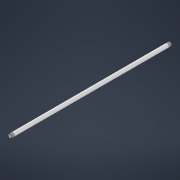
# Autodesk Inventor part: Welle
Saved by Autodesk Inventor 2021 (Build 250183000, 183)
## iProperties
Created: 2023-10-25
Part Number: Welle
Material: Generisch
Document SubType Name: Modeling
Designer: Tobias Sauter
Density: 1 g/cm^3
Appearance: Vorgabe
Author: Team 8
Autodesk Inventor part; units mm, degrees
ref_plane "YZ Plane" through (0, 0, 0) normal (1, 0, 0) x (0, 1, 0)
ref_plane "XZ Plane" through (0, 0, 0) normal (0, 1, 0) x (-1, 0, 0)
ref_plane "XY Plane" through (0, 0, 0) normal (0, 0, 1) x (1, 0, 0)
sketch "Skizze1" plane through (0, 0, 0) normal (0, 0, 1) x (1, 0, 0)
  circle A0 centre (0, 0) radius 2.5
  dimension "d0" = 5
  constraints: 1 centre point, 1 coincident
  measures "d0" diameter of A0
extrude "Extrusion1" add sketch "Skizze1" along normal blind 215
thread "Gewinde1" size "M5x0.8" class "6g" standard "ISO Metric profile" length 4.2
thread "Gewinde2" size "M5x0.8" class "6g" standard "ISO Metric profile" length 4.2
